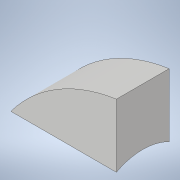
# Autodesk Inventor part: picameraholder
Saved by Autodesk Inventor 2020.3 (Build 243373000, 373)
## iProperties
Created: 2021-04-28
Part Number: picameraholder
Material: Generic
Document SubType Name: Modeling
Designer: kibandi
Mass: 21.9168 g
Surface Area: 53.4601 cm^2
Volume: 21.9168 cm^3
Density: 1 g/cm^3
Appearance: Default
Author: kibandi
Autodesk Inventor part; units mm, degrees
ref_plane "YZ Plane" through (0, 0, 0) normal (1, 0, 0) x (0, 1, 0)
ref_plane "XZ Plane" through (0, 0, 0) normal (0, 1, 0) x (-1, 0, 0)
ref_plane "XY Plane" through (0, 0, 0) normal (0, 0, 1) x (1, 0, 0)
sketch "Sketch1" plane through (0, 0, 0) normal (1, 0, 0) x (0, 1, 0)
  arc A0 (23.7063, -12.5) -> (23.7063, 12.5) centre (0, 0) ccw
  line L0 (23.7063, 12.5) -> (53.7063, 12.5)
  line L1 (53.7063, 12.5) -> (53.7063, -12.5)
  line L2 (53.7063, -12.5) -> (23.7063, -12.5)
  line L3 (23.7063, 12.5) -> (23.7063, -12.5)
  dimension "d0" = 53.6
  dimension "d3" = 30
  dimension "d4" = 25
  dimension "d5" = 26.8
  constraints: 8 end point, 2 point on circle, 1 centre point, 1 coincident, 1 perpendicular, 1 vertical
  measures "d0" diameter of A0
  measures "d3" distance of L0.start L0.end
  measures "d4" distance of L0.end L1.end
  measures "d5" radius of A0
extrude "Extrusion1" add sketch "Sketch1" against normal blind 50 contours A0 L0 L1 L2
sketch "Sketch2" plane through (0, 23.7063, 12.5) normal (0, 0, 1) x (1, 0, 0)
  line L0 (0, 30) -> (0, 0) projected
  line L1 (-50, 0) -> (-50, 3.0937) projected
  arc A0 (0, 30) -> (-50, 0) centre (10.8981, -44.8302) ccw
  line L2 (0, 30) -> (-50, 30) projected
  line L3 (0, 30) -> (-50, 30)
  line L4 (0, 0) -> (-50, 0) projected
  line L5 (-50, 30) -> (-50, 0)
  point P0 (0, -23.7063)
  constraints: 4 end point, 2 point on circle, 1 centre point, 1 collinear, 1 perpendicular
extrude "Extrusion2" cut sketch "Sketch2" against normal blind 25 contours A0 L1 L5 L2
body "Solid1"
